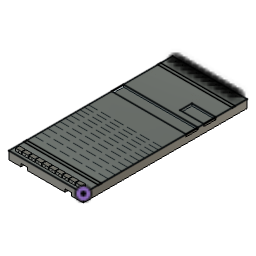
HarpejjiBody (Autodesk Fusion 360 design; units mm, degrees)
Autodesk Fusion 360 part; units mm, degrees
sketch "Sketch1" plane through (0, 0, 0) normal (0, 0, 1) x (1, 0, 0)
  line L0 (0, 0) -> (-250, 0)
  line L1 (-250, 0) -> (-250, 550)
  line L2 (-250, 550) -> (0, 550)
  line L3 (0, 550) -> (0, 0)
  line L4 (-250, 385) -> (0, 385)
  line L5 (0, 385) -> (0, 345)
  line L6 (0, 345) -> (-250, 345)
  line L7 (-250, 345) -> (-250, 385)
  line L8 (-250, 60) -> (0, 60)
  line L9 (0, 60) -> (0, 50)
  line L10 (0, 50) -> (-250, 50)
  line L11 (-250, 50) -> (-250, 60)
  line L12 (-250, 510) -> (0, 510)
  line L13 (0, 510) -> (0, 500)
  line L14 (0, 500) -> (-250, 500)
  line L15 (-250, 500) -> (-250, 510)
  line L16 (-250, 84.695) -> (0, 84.695) construction
  line L17 (-250, 108.004) -> (0, 108.004) construction
  line L18 (-250, 130.005) -> (0, 130.005) construction
  line L19 (-250, 150.771) -> (0, 150.771) construction
  line L20 (-250, 170.372) -> (0, 170.372) construction
  line L21 (-250, 188.873) -> (0, 188.873) construction
  line L22 (-250, 206.335) -> (0, 206.335) construction
  line L23 (-250, 222.817) -> (0, 222.817) construction
  line L24 (-250, 238.374) -> (0, 238.374) construction
  line L25 (-250, 253.058) -> (0, 253.058) construction
  line L26 (-250, 266.918) -> (0, 266.918) construction
  line L27 (0, 445) -> (-80, 445)
  line L28 (-80, 445) -> (-80, 405)
  line L29 (-80, 405) -> (0, 405)
  line L30 (0, 405) -> (0, 445)
  point P0 (-229, 540)
  point P1 (-206.5, 540)
  point P2 (-184, 540)
  point P3 (-161.5, 540)
  point P4 (-139, 540)
  point P5 (-116.5, 540)
  point P6 (-94, 540)
  point P7 (-71.5, 540)
  point P8 (-49, 540)
  point P9 (-26.5, 540)
  dimension "d1" = 250
  dimension "d2" = 550
  dimension "d3" = 21
  dimension "d6" = 22.5
  dimension "d7" = -525
  dimension "d41" = 10
  dimension "d42" = 165
  dimension "d43" = 40
  dimension "d44" = 60
  dimension "d45" = 10
  dimension "d46" = 40
  dimension "d47" = 10
  dimension "d48" = 24.695
  dimension "d49" = 23.309
  dimension "d50" = 22.001
  dimension "d51" = 20.766
  dimension "d52" = 19.601
  dimension "d53" = 18.501
  dimension "d54" = 17.462
  dimension "d55" = 16.482
  dimension "d56" = 15.557
  dimension "d57" = 14.684
  dimension "d58" = 13.86
  dimension "d60" = 20
  dimension "d61" = 40
  dimension "d62" = 80
  constraint horizontal L0
  constraint vertical L1
  constraint horizontal L2
  constraint vertical L3
  constraint coincident L0.start L3.end
  constraint horizontal L4
  constraint vertical L5
  constraint horizontal L6
  constraint vertical L7
  constraint coincident L3 L5.end
  constraint coincident L1 L4.start
  constraint horizontal L8
  constraint vertical L9
  constraint horizontal L10
  constraint vertical L11
  constraint coincident L3 L9.end
  constraint coincident L1 L8.start
  constraint horizontal L12
  constraint vertical L13
  constraint horizontal L14
  constraint vertical L15
  constraint coincident L3 L13.end
  constraint coincident L1 L12.start
  constraint coincident L1 L16.start
  constraint coincident L3 L16.end
  constraint perpendicular L3 L16
  constraint coincident L1 L17.start
  constraint coincident L3 L17.end
  constraint perpendicular L3 L17
  constraint coincident L1 L18.start
  constraint coincident L3 L18.end
  constraint perpendicular L3 L18
  constraint coincident L1 L19.start
  constraint coincident L3 L19.end
  constraint perpendicular L3 L19
  constraint coincident L1 L20.start
  constraint coincident L3 L20.end
  constraint perpendicular L3 L20
  constraint coincident L1 L21.start
  constraint coincident L3 L21.end
  constraint perpendicular L3 L21
  constraint coincident L1 L22.start
  constraint coincident L3 L22.end
  constraint perpendicular L3 L22
  constraint coincident L1 L23.start
  constraint coincident L3 L23.end
  constraint perpendicular L3 L23
  constraint coincident L1 L24.start
  constraint coincident L3 L24.end
  constraint perpendicular L3 L24
  constraint coincident L1 L25.start
  constraint coincident L3 L25.end
  constraint perpendicular L3 L25
  constraint coincident L1 L26.start
  constraint coincident L3 L26.end
  constraint perpendicular L3 L26
  constraint horizontal L27
  constraint vertical L28
  constraint horizontal L29
  constraint vertical L30
  constraint coincident L3 L27.start
  measures "d1" distance of L1.end L2.end
  measures "d2" distance of L0.start L2.end
  measures "d3" distance of L1 P0
  measures "d41" distance of L2 P0
  measures "d42" distance of L2 L4
  measures "d43" distance of L4 L6
  measures "d44" distance of L0 L8
  measures "d45" distance of L8 L10
  measures "d46" distance of L2 L12
  measures "d47" distance of L12 L14
  measures "d48" distance of L8 L16
  measures "d49" distance of L16 L17
  measures "d50" distance of L17 L18
  measures "d51" distance of L18 L19
  measures "d52" distance of L19 L20
  measures "d53" distance of L20 L21
  measures "d54" distance of L21 L22
  measures "d55" distance of L22 L23
  measures "d56" distance of L23 L24
  measures "d57" distance of L24 L25
  measures "d58" distance of L25 L26
  measures "d60" distance of L4 L29
  measures "d61" distance of L27 L29
  measures "d62" distance of L3 L28
extrude "Extrude1" add sketch "Sketch1" against normal blind 27 makes body 1
extrude "Extrude5" cut sketch "Sketch1" against normal blind 7.5 contours L1 L3 L4 L5 L6 L7 | L3 L27 L28 L29 L30 bodies 1
hole "Hole2" at (-229, 540, 0) at (-206.5, 540, 0) at (-184, 540, 0) at (-161.5, 540, 0) at (-139, 540, 0) at (-116.5, 540, 0) at (-94, 540, 0) at (-71.5, 540, 0) at (-49, 540, 0) at (-26.5, 540, 0) direction (0, 0, -1) diameter 3 depth 1000 tip angle 118 bodies 1
sketch "Sketch1 (2)" plane through (0, 0, 0) normal (0, 0, 1) x (1, 0, 0) in component "bridge piece"
  line L0 (0, 0) -> (20, 0)
  line L1 (20, 0) -> (20, 13)
  line L2 (20, 13) -> (0, 13)
  line L3 (0, 13) -> (0, 0)
  dimension "d69" = 20
  dimension "d70" = 13
  constraint horizontal L0
  constraint vertical L1
  constraint horizontal L2
  constraint vertical L3
  constraint coincident L0.start L3.end
  measures "d69" distance of L0.start L0.end
  measures "d70" distance of L0.end L1.end
extrude "Extrude1'" add sketch "Sketch1 (2)" along normal blind 9 separate body makes body 2 in component "bridge piece"
sketch "Sketch2" plane through (0, 0, 0) normal (0, -1, 0) x (1, 0, 0) in component "bridge piece"
  line L0 (0, 0) -> (20, 0)
  line L1 (20, 0) -> (20, 9)
  line L2 (20, 9) -> (0, 9)
  line L3 (0, 9) -> (0, 0)
  point P0 (10, 4.5)
  dimension "d73" = 4.5
  dimension "d74" = 10
  measures "d73" distance of L2 P0
  measures "d74" distance of L3 P0
hole "Hole1" at (10, 0, 4.5) direction (0, 1, 0) diameter 2 depth 100 tip angle 118 bodies 2 in component "bridge piece"
sketch "Sketch4" plane through (0, 0, 0) normal (0, 0, 1) x (1, 0, 0)
  line L0 (-227.5, 540) -> (-227.5, 16) construction
  circle A0 centre (-229, 540) radius 1.5
  point P0 (-227.5, 16)
  point P1 (-205, 16)
  point P2 (-182.5, 16)
  point P3 (-160, 16)
  point P4 (-137.5, 16)
  point P5 (-115, 16)
  point P6 (-92.5, 16)
  point P7 (-70, 16)
  point P8 (-47.5, 16)
  point P9 (-25, 16)
  dimension "d78" = 524
  dimension "d81" = 22.5
  dimension "d82" = 0
  constraint vertical L0
  constraint tangent L0 A0
  constraint coincident P0 L0.end
  measures "d78" distance of L0.start P0
pattern_linear "R-Pattern1" count 10 spacing 22.5 along (1, 0, 0) of bodies 2 makes body 3 at (29.1667, 8.6667, 0) makes body 4 at (51.6667, 8.6667, 0) makes body 5 at (74.1667, 8.6667, 0) makes body 6 at (96.6667, 8.6667, 0) makes body 7 at (119.1667, 8.6667, 0) makes body 8 at (141.6667, 8.6667, 0) makes body 9 at (164.1667, 8.6667, 0) makes body 10 at (186.6667, 8.6667, 0) makes body 11 at (209.1667, 8.6667, 0) in component "bridge piece"
sketch "Sketch5" plane through (0, 0, -27) normal (0, 0, -1) x (1, 0, 0)
  circle A0 centre (-49, -540) radius 1.5
  circle A1 centre (-94, -540) radius 1.5
  circle A2 centre (-139, -540) radius 1.5
  circle A3 centre (-184, -540) radius 1.5
  circle A4 centre (-229, -540) radius 1.5
  circle A5 centre (-206.5, -540) radius 1.5
  circle A6 centre (-161.5, -540) radius 1.5
  circle A7 centre (-116.5, -540) radius 1.5
  circle A8 centre (-71.5, -540) radius 1.5
  circle A9 centre (-26.5, -540) radius 1.5
  line L0 (0, -550) -> (0, 0)
  line L1 (0, 0) -> (-250, 0)
  line L2 (-250, 0) -> (-250, -550)
  line L3 (-250, -550) -> (0, -550)
  line L4 (-210, 0) -> (-188, 0)
  line L5 (-188, 0) -> (-188, -518)
  line L6 (-188, -518) -> (-210, -518)
  line L7 (-210, -518) -> (-210, 0)
  line L8 (-62, 0) -> (-40, 0)
  line L9 (-40, 0) -> (-40, -518)
  line L10 (-40, -518) -> (-62, -518)
  line L11 (-62, -518) -> (-62, 0)
  dimension "d87" = 40
  dimension "d88" = 22
  dimension "d89" = 518
  dimension "d90" = 40
  constraint horizontal L4
  constraint vertical L5
  constraint horizontal L6
  constraint vertical L7
  constraint coincident L1 L4.start
  constraint horizontal L8
  constraint vertical L9
  constraint horizontal L10
  constraint vertical L11
  constraint coincident L1 L8.start
  constraint equal L7 L11
  constraint equal L6 L10
  measures "d87" distance of L2 L7
  measures "d88" distance of L5 L7
  measures "d89" distance of L4.start L6.end
  measures "d90" distance of L0 L9
extrude "Extrude6" cut sketch "Sketch5" against normal blind 10 contours L1 L8 L9 L10 L11 | L1 L4 L5 L6 L7 bodies 1
component "bridge piece" placed x (1, 0, 0) y (0, 1, 0) z (0, 0, 1) at (-237.5, 9.5, 0)
component "Component" placed x (1, 0, 0) y (0, 1, 0) z (0, 0, 1) at (257.0542, 5.3782, 0) in component "bridge piece"
